Autodesk Inventor part; units mm, degrees
(part 2 of 2)
sketch "Sketch23 outline for RSAHolderHex" plane through (0, -10, 0) normal (0, -1, 0) x (1, 0, 0)
  line L0 (7.80058, -8.259557) -> (9.35908, -10.958958)
  line L1 (9.35908, -5.560156) -> (7.80058, -8.259557)
  line L2 (12.47608, -5.560156) -> (9.35908, -5.560156)
  line L3 (14.03458, -8.259557) -> (12.47608, -5.560156)
  line L4 (12.47608, -10.958958) -> (14.03458, -8.259557)
  line L5 (9.35908, -10.958958) -> (12.47608, -10.958958)
  line L6 (14.208131, -11.958958) -> (15.766631, -14.65836)
  line L7 (15.766631, -9.259557) -> (14.208131, -11.958958)
  line L8 (18.883631, -9.259557) -> (15.766631, -9.259557)
  line L9 (20.442131, -11.958958) -> (18.883631, -9.259557)
  line L10 (18.883631, -14.65836) -> (20.442131, -11.958958)
  line L11 (15.766631, -14.65836) -> (18.883631, -14.65836)
  line L12 (18.883631, -1.860755) -> (15.766631, -1.860755)
  line L13 (20.442131, -4.560156) -> (18.883631, -1.860755)
  line L14 (18.883631, -7.259557) -> (20.442131, -4.560156)
  line L15 (15.766631, -7.259557) -> (18.883631, -7.259557)
  line L16 (14.208131, -4.560156) -> (15.766631, -7.259557)
  line L17 (15.766631, -1.860755) -> (14.208131, -4.560156)
  line L18 (31.698732, -14.65836) -> (33.257232, -11.958958)
  line L19 (28.581732, -14.65836) -> (31.698732, -14.65836)
  line L20 (27.023232, -11.958958) -> (28.581732, -14.65836)
  line L21 (28.19275, -9.933295) -> (27.023232, -11.958958)
  line L22 (32.087715, -9.933295) -> (28.19275, -9.933295)
  line L23 (33.257232, -11.958958) -> (32.087715, -9.933295)
  line L24 (38.106283, -12.958958) -> (34.989283, -12.958958)
  line L25 (39.273785, -14.981131) -> (38.106283, -12.958958)
  line L26 (33.814917, -14.99302) -> (39.273785, -14.981131)
  line L27 (34.989283, -12.958958) -> (33.814917, -14.99302)
  line L28 (34.989283, -10.958958) -> (38.106283, -10.958958)
  line L29 (34.397116, -9.933295) -> (34.989283, -10.958958)
  line L30 (38.69845, -9.933295) -> (34.397116, -9.933295)
  line L31 (38.106283, -10.958958) -> (38.69845, -9.933295)
  line L32 (44.513834, -14.65836) -> (46.072334, -11.958958)
  line L33 (41.396834, -14.65836) -> (44.513834, -14.65836)
  line L34 (39.838334, -11.958958) -> (41.396834, -14.65836)
  line L35 (41.007851, -9.933295) -> (39.838334, -11.958958)
  line L36 (44.902816, -9.933295) -> (41.007851, -9.933295)
  line L37 (46.072334, -11.958958) -> (44.902816, -9.933295)
  line L38 (50.921385, -12.958958) -> (47.804385, -12.958958)
  line L39 (52.072793, -14.953256) -> (50.921385, -12.958958)
  line L40 (46.646153, -14.965075) -> (52.072793, -14.953256)
  line L41 (47.804385, -12.958958) -> (46.646153, -14.965075)
  line L42 (47.804385, -10.958958) -> (50.921385, -10.958958)
  line L43 (47.212217, -9.933295) -> (47.804385, -10.958958)
  line L44 (51.513552, -9.933295) -> (47.212217, -9.933295)
  line L45 (50.921385, -10.958958) -> (51.513552, -9.933295)
  line L46 (58.887435, -11.958958) -> (57.328935, -9.259557)
  line L47 (57.328935, -14.65836) -> (58.887435, -11.958958)
  line L48 (54.211935, -14.65836) -> (57.328935, -14.65836)
  line L49 (52.653435, -11.958958) -> (54.211935, -14.65836)
  line L50 (53.822953, -9.933295) -> (52.653435, -11.958958)
  line L51 (56.238399, -9.933295) -> (53.822953, -9.933295)
  line L52 (56.238399, -9.259557) -> (56.238399, -9.933295)
  line L53 (57.328935, -9.259557) -> (56.238399, -9.259557)
  line L54 (60.619486, -5.560156) -> (59.060986, -8.259557)
  line L55 (61.238399, -5.560156) -> (60.619486, -5.560156)
  line L56 (61.238399, -10.958958) -> (61.238399, -5.560156)
  line L57 (60.619486, -10.958958) -> (61.238399, -10.958958)
  line L58 (59.060986, -8.259557) -> (60.619486, -10.958958)
  line L59 (58.887435, -4.560156) -> (57.328935, -1.860755)
  line L60 (57.328935, -7.259557) -> (58.887435, -4.560156)
  line L61 (56.238399, -7.259557) -> (57.328935, -7.259557)
  line L62 (56.238399, -1.860755) -> (56.238399, -7.259557)
  line L63 (57.328935, -1.860755) -> (56.238399, -1.860755)
  line L64 (61.238399, 3.838646) -> (61.238399, 5.566705)
  line L65 (61.238399, 5.566705) -> (59.621791, 5.566705)
  line L66 (59.621791, 5.566705) -> (60.619486, 3.838646)
  line L67 (60.619486, 3.838646) -> (61.238399, 3.838646)
  line L68 (60.619486, 1.838646) -> (59.060986, -0.860755)
  line L69 (61.238399, 1.838646) -> (60.619486, 1.838646)
  line L70 (61.238399, -3.560156) -> (61.238399, 1.838646)
  line L71 (60.619486, -3.560156) -> (61.238399, -3.560156)
  line L72 (59.060986, -0.860755) -> (60.619486, -3.560156)
  line L73 (57.328935, 0.139245) -> (58.887435, 2.838646)
  line L74 (56.238399, 0.139245) -> (57.328935, 0.139245)
  line L75 (56.238399, 0.566705) -> (56.238399, 0.139245)
  line L76 (53.965141, 0.566705) -> (56.238399, 0.566705)
  line L77 (52.653435, 2.838646) -> (53.965141, 0.566705)
  line L78 (54.211935, 5.538047) -> (52.653435, 2.838646)
  line L79 (57.328935, 5.538047) -> (54.211935, 5.538047)
  line L80 (58.887435, 2.838646) -> (57.328935, 5.538047)
  line L81 (50.921385, 1.838646) -> (47.804385, 1.838646)
  line L82 (51.65574, 0.566705) -> (50.921385, 1.838646)
  line L83 (47.070029, 0.566705) -> (51.65574, 0.566705)
  line L84 (47.804385, 1.838646) -> (47.070029, 0.566705)
  line L85 (47.804385, 3.838646) -> (50.921385, 3.838646)
  line L86 (46.806689, 5.566705) -> (47.804385, 3.838646)
  line L87 (51.91908, 5.566705) -> (46.806689, 5.566705)
  line L88 (50.921385, 3.838646) -> (51.91908, 5.566705)
  line L89 (41.396834, 5.538047) -> (39.838334, 2.838646)
  line L90 (44.513834, 5.538047) -> (41.396834, 5.538047)
  line L91 (46.072334, 2.838646) -> (44.513834, 5.538047)
  line L92 (44.760628, 0.566705) -> (46.072334, 2.838646)
  line L93 (41.150039, 0.566705) -> (44.760628, 0.566705)
  line L94 (39.838334, 2.838646) -> (41.150039, 0.566705)
  line L95 (38.106283, 1.838646) -> (34.989283, 1.838646)
  line L96 (38.840638, 0.566705) -> (38.106283, 1.838646)
  line L97 (34.254928, 0.566705) -> (38.840638, 0.566705)
  line L98 (34.989283, 1.838646) -> (34.254928, 0.566705)
  line L99 (34.989283, 3.838646) -> (38.106283, 3.838646)
  line L100 (33.991588, 5.566705) -> (34.989283, 3.838646)
  line L101 (39.103978, 5.566705) -> (33.991588, 5.566705)
  line L102 (38.106283, 3.838646) -> (39.103978, 5.566705)
  line L103 (31.698732, 5.538047) -> (28.581732, 5.538047)
  line L104 (33.257232, 2.838646) -> (31.698732, 5.538047)
  line L105 (31.945526, 0.566705) -> (33.257232, 2.838646)
  line L106 (28.334938, 0.566705) -> (31.945526, 0.566705)
  line L107 (27.023232, 2.838646) -> (28.334938, 0.566705)
  line L108 (28.581732, 5.538047) -> (27.023232, 2.838646)
  line L109 (22.174181, 3.838646) -> (25.291181, 3.838646)
  line L110 (20.615681, 6.538047) -> (22.174181, 3.838646)
  line L111 (21.924267, 8.804584) -> (20.615681, 6.538047)
  arc A0 (25.827358, 5.488791) -> (21.924267, 8.804584) centre (13.936454, -4.553147) ccw
  line L112 (26.243893, 5.488791) -> (25.827358, 5.488791)
  line L113 (25.291181, 3.838646) -> (26.243893, 5.488791)
  line L114 (15.766631, 7.538047) -> (18.883631, 7.538047)
  line L115 (14.208131, 10.237449) -> (15.766631, 7.538047)
  line L116 (14.489622, 10.725006) -> (14.208131, 10.237449)
  arc A1 (19.994829, 9.4627) -> (14.489622, 10.725006) centre (13.836061, -4.761209) ccw
  line L117 (18.883631, 7.538047) -> (19.994829, 9.4627)
  line L118 (7.80058, 6.538047) -> (9.35908, 3.838646)
  line L119 (9.35908, 9.237449) -> (7.80058, 6.538047)
  line L120 (12.47608, 9.237449) -> (9.35908, 9.237449)
  line L121 (14.03458, 6.538047) -> (12.47608, 9.237449)
  line L122 (12.47608, 3.838646) -> (14.03458, 6.538047)
  line L123 (9.35908, 3.838646) -> (12.47608, 3.838646)
  line L124 (1.393029, 2.838646) -> (2.951529, 0.139245)
  line L125 (2.951529, 5.538047) -> (1.393029, 2.838646)
  line L126 (6.068529, 5.538047) -> (2.951529, 5.538047)
  line L127 (7.627029, 2.838646) -> (6.068529, 5.538047)
  line L128 (6.068529, 0.139245) -> (7.627029, 2.838646)
  line L129 (2.951529, 0.139245) -> (6.068529, 0.139245)
  line L130 (1.219478, -8.259557) -> (-0.339022, -5.560156)
  line L131 (-0.287781, -10.870207) -> (1.219478, -8.259557)
  arc A2 (-1.594806, -5.560156) -> (-0.287781, -10.870207) centre (13.936454, -4.553147) ccw
  line L132 (-0.339022, -5.560156) -> (-1.594806, -5.560156)
  line L133 (-0.339022, -3.560156) -> (1.219478, -0.860755)
  line L134 (-1.595709, -3.560156) -> (-0.339022, -3.560156)
  arc A3 (-1.422914, -2.038404) -> (-1.595709, -3.560156) centre (13.936454, -4.553147) ccw
  arc A4 (-0.255666, 1.69427) -> (-1.422914, -2.038404) centre (13.836061, -4.761209) ccw
  line L135 (1.219478, -0.860755) -> (-0.255666, 1.69427)
  line L136 (2.951529, -1.860755) -> (1.393029, -4.560156)
  line L137 (6.068529, -1.860755) -> (2.951529, -1.860755)
  line L138 (7.627029, -4.560156) -> (6.068529, -1.860755)
  line L139 (6.068529, -7.259557) -> (7.627029, -4.560156)
  line L140 (2.951529, -7.259557) -> (6.068529, -7.259557)
  line L141 (1.393029, -4.560156) -> (2.951529, -7.259557)
  arc A5 (4.153922, -16.65836) -> (7.172415, -18.570347) centre (13.936454, -4.553147) ccw
  line L142 (6.068529, -16.65836) -> (4.153922, -16.65836)
  line L143 (7.172415, -18.570347) -> (6.068529, -16.65836)
  line L144 (2.951529, -14.65836) -> (6.068529, -14.65836)
  line L145 (1.393029, -11.958958) -> (2.951529, -14.65836)
  line L146 (2.951529, -9.259557) -> (1.393029, -11.958958)
  line L147 (6.068529, -9.259557) -> (2.951529, -9.259557)
  line L148 (7.627029, -11.958958) -> (6.068529, -9.259557)
  line L149 (6.068529, -14.65836) -> (7.627029, -11.958958)
  line L150 (7.80058, -15.65836) -> (9.35908, -18.357761)
  line L151 (9.35908, -12.958958) -> (7.80058, -15.65836)
  line L152 (12.47608, -12.958958) -> (9.35908, -12.958958)
  line L153 (14.03458, -15.65836) -> (12.47608, -12.958958)
  line L154 (12.47608, -18.357761) -> (14.03458, -15.65836)
  line L155 (9.35908, -18.357761) -> (12.47608, -18.357761)
  line L156 (15.766631, -16.65836) -> (14.208131, -19.357761)
  line L157 (18.883631, -16.65836) -> (15.766631, -16.65836)
  line L158 (20.136676, -18.828698) -> (18.883631, -16.65836)
  arc A6 (14.637371, -20.101228) -> (20.136676, -18.828698) centre (13.936454, -4.553147) ccw
  line L159 (14.208131, -19.357761) -> (14.637371, -20.101228)
  line L160 (25.291181, -12.958958) -> (22.174181, -12.958958)
  line L161 (26.474777, -15.009006) -> (25.291181, -12.958958)
  line L162 (25.463077, -15.011209) -> (26.474777, -15.009006)
  arc A7 (21.918249, -17.914474) -> (25.463077, -15.011209) centre (13.936454, -4.553147) ccw
  line L163 (20.615681, -15.65836) -> (21.918249, -17.914474)
  line L164 (22.174181, -12.958958) -> (20.615681, -15.65836)
  line L165 (22.174181, -10.958958) -> (25.291181, -10.958958)
  line L166 (20.615681, -8.259557) -> (22.174181, -10.958958)
  line L167 (22.174181, -5.560156) -> (20.615681, -8.259557)
  line L168 (25.291181, -5.560156) -> (22.174181, -5.560156)
  line L169 (26.849681, -8.259557) -> (25.291181, -5.560156)
  line L170 (25.291181, -10.958958) -> (26.849681, -8.259557)
  line L171 (25.291181, 1.838646) -> (22.174181, 1.838646)
  line L172 (26.849681, -0.860755) -> (25.291181, 1.838646)
  line L173 (25.291181, -3.560156) -> (26.849681, -0.860755)
  line L174 (22.174181, -3.560156) -> (25.291181, -3.560156)
  line L175 (20.615681, -0.860755) -> (22.174181, -3.560156)
  line L176 (22.174181, 1.838646) -> (20.615681, -0.860755)
  line L177 (15.766631, 0.139245) -> (18.883631, 0.139245)
  line L178 (14.208131, 2.838646) -> (15.766631, 0.139245)
  line L179 (15.766631, 5.538047) -> (14.208131, 2.838646)
  line L180 (18.883631, 5.538047) -> (15.766631, 5.538047)
  line L181 (20.442131, 2.838646) -> (18.883631, 5.538047)
  line L182 (18.883631, 0.139245) -> (20.442131, 2.838646)
  line L183 (7.80058, -0.860755) -> (9.35908, -3.560156)
  line L184 (9.35908, 1.838646) -> (7.80058, -0.860755)
  line L185 (12.47608, 1.838646) -> (9.35908, 1.838646)
  line L186 (14.03458, -0.860755) -> (12.47608, 1.838646)
  line L187 (12.47608, -3.560156) -> (14.03458, -0.860755)
  line L188 (9.35908, -3.560156) -> (12.47608, -3.560156)
  arc A8 (7.18363, 9.46946) -> (4.1366, 7.538047) centre (13.936454, -4.553147) ccw
  line L189 (6.068529, 7.538047) -> (7.18363, 9.46946)
  line L190 (4.1366, 7.538047) -> (6.068529, 7.538047)
  line L191 (6.068529, 12.93685) -> (2.951529, 12.93685)
  line L192 (7.213176, 10.954264) -> (6.068529, 12.93685)
  arc A9 (2.651998, 8.056851) -> (7.213176, 10.954264) centre (13.932065, -4.661643) cw
  line L193 (1.393029, 10.237449) -> (2.651998, 8.056851)
  line L194 (2.951529, 12.93685) -> (1.393029, 10.237449)
extrude "RSAHolderHex" cut sketch "Sketch23 outline for RSAHolderHex" against normal blind 10
equation "\"d89\" = d19"
body "Solid3"
